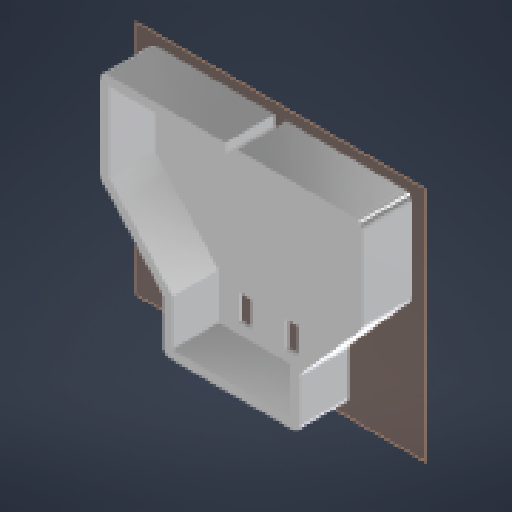
# Autodesk Inventor part: kracken Cover
Saved by Autodesk Inventor 2023 (Build 270158000, 158)
## iProperties
Created: 2024-02-18
Part Number: kracken Cover
Material: Aluminum 6061
Document SubType Name: Modeling
Designer: mavericks
Density: 2.7 g/cm^3
Appearance: Aluminum - Flat
Author: mavericks
Autodesk Inventor part; units mm, degrees
ref_plane "YZ Plane" through (0, 0, 0) normal (1, 0, 0) x (0, 1, 0)
ref_plane "XZ Plane" through (0, 0, 0) normal (0, 1, 0) x (-1, 0, 0)
ref_plane "Work Plane1" through (0, 0, -5.08) normal (0, 0, 1) x (1, 0, 0)
sketch "Sketch1" plane through (0, 0, -5.08) normal (0, 0, 1) x (1, 0, 0)
  line L0 (20.772, 33.401) -> (20.772, 19.8332)
  line L1 (20.772, 33.401) -> (1.011, 33.401)
  line L2 (1.011, 33.401) -> (1.011, 27.686)
  line L3 (1.011, 27.686) -> (-1.011, 27.686)
  line L4 (-1.011, 27.686) -> (-1.011, 33.401)
  line L5 (-1.011, 33.401) -> (-20.772, 33.401)
  line L6 (-20.772, 33.401) -> (-20.772, 19.8332)
  line L7 (-20.772, 19.8332) -> (-10.033, 7.78)
  line L8 (-10.033, 7.78) -> (-10.033, 0)
  line L9 (-10.033, 0) -> (10.033, 0)
  line L10 (10.033, 0) -> (10.033, 7.78)
  line L11 (10.033, 7.78) -> (20.772, 19.8332)
  line L12 (-22.3595, 34.9885) -> (-0.5765, 34.9885)
  line L13 (-0.5765, 34.9885) -> (22.3595, 34.9885)
  line L14 (22.3595, 34.9885) -> (22.3595, 19.2286)
  line L15 (22.3595, 19.2286) -> (11.6205, 7.1754)
  line L16 (11.6205, 7.1754) -> (11.6205, -1.5875)
  line L17 (11.6205, -1.5875) -> (-11.6205, -1.5875)
  line L18 (-11.6205, -1.5875) -> (-11.6205, 7.1754)
  line L19 (-11.6205, 7.1754) -> (-22.3595, 19.2286)
  line L20 (-22.3595, 19.2286) -> (-22.3595, 34.9885)
  point P0 (0, 0)
  point P1 (0, 0)
  point P2 (0, 27.686)
  point P3 (0, 0)
  dimension "d1" = 41.544
  dimension "d2" = 19.761
  dimension "d3" = 19.761
  dimension "d6" = 20.066
  dimension "d7" = 138.3
  dimension "d8" = 138.3
  dimension "d9" = 33.401
  dimension "d10" = 5.715
  dimension "d11" = 25.621
  dimension "d12" = 1.5875
  constraints: 42 end point, 9 perpendicular, 4 coincident, 2 midpoint, 2 point on line, 1 horizontal, 1 horizontal alignment, 1 vertical, 1 vertical alignment, 8 other
  measures "d1" distance between parallel lines of L0 L6
  measures "d2" distance of L4.end L5.end
  measures "d3" distance of L0.start L1.end
  measures "d6" distance of L8.end L9.end
  measures "d7" angle of L7 L6
  measures "d8" angle of L11 L0
  measures "d9" distance between parallel lines of L9 L5
  measures "d10" distance between parallel lines of L3 L5
  measures "d11" distance from line of L7.end L5
  measures "d12" distance between parallel lines of L5 L12
extrude "Extrusion1" add sketch "Sketch1" along normal blind 8.382
extrude "Extrusion2" add sketch "Sketch1" along normal blind 0.508 contours L0 L11 L10 L9 L8 L7 L6 L5 L4 L3 L2 L1
sketch "Sketch2" plane through (0, 0, 3.302) normal (0, 0, 1) x (1, 0, 0)
  line L0 (-22.3595, 34.9885) -> (22.3595, 34.9885) construction
  line L1 (-1.011, 27.686) -> (1.011, 27.686)
  line L2 (1.011, 27.686) -> (1.011, 34.9885)
  line L3 (1.011, 34.9885) -> (-1.011, 34.9885)
  line L4 (-1.011, 34.9885) -> (-1.011, 27.686)
  point P0 (0, 0)
  constraints: 8 end point, 2 parallel, 1 horizontal, 1 perpendicular, 1 point on line
extrude "Extrusion3" cut sketch "Sketch2" against normal through all
fillet "Fillet1" radius 1.27 8 edges at (-22.3595, 34.9885, -0.889) (-22.3595, 19.2286, -0.889) (-11.6205, 7.1754, -0.889) (-11.6205, -1.5875, -0.889) (11.6205, -1.5875, -0.889) (11.6205, 7.1754, -0.889) (22.3595, 19.2286, -0.889) (22.3595, 34.9885, -0.889)
sketch "Sketch4" plane through (0, 0, -5.08) normal (0, 0, -1) x (-1, 0, 0)
  circle A0 centre (-14.2442, 29.337) radius 1.8288 construction
  circle A1 centre (14.2546, 29.337) radius 1.8288 construction
  circle A2 centre (-14.2442, 29.337) radius 3.81
  circle A3 centre (14.2546, 29.337) radius 3.81
  line L0 (-1.8894, 5.6982) -> (-2.9308, 5.6982) construction
  line L1 (-2.9308, 2.3282) -> (-2.9308, 5.6982) construction
  line L2 (-2.9308, 2.3282) -> (-1.8894, 2.3282) construction
  line L3 (-1.8894, 5.6982) -> (-1.8894, 2.3282) construction
  line L4 (6.0354, 5.6982) -> (4.994, 5.6982) construction
  line L5 (4.994, 2.3282) -> (4.994, 5.6982) construction
  line L6 (4.994, 2.3282) -> (6.0354, 2.3282) construction
  line L7 (6.0354, 5.6982) -> (6.0354, 2.3282) construction
  line L8 (-1.3814, 1.8202) -> (-3.4388, 1.8202)
  line L9 (-3.4388, 1.8202) -> (-3.4388, 6.2062)
  line L10 (-3.4388, 6.2062) -> (-1.3814, 6.2062)
  line L11 (-1.3814, 6.2062) -> (-1.3814, 1.8202)
  line L12 (4.486, 6.2062) -> (6.5434, 6.2062)
  line L13 (6.5434, 6.2062) -> (6.5434, 1.8202)
  line L14 (6.5434, 1.8202) -> (4.486, 1.8202)
  line L15 (4.486, 1.8202) -> (4.486, 6.2062)
  point P0 (0, 0)
  dimension "d30" = 7.62
  dimension "d33" = 0.508
  dimension "d34" = 0.508
  constraints: 16 end point, 2 centre point, 2 coincident, 1 equal radius, 6 other
  measures "d30" diameter of A2
  measures "d33" distance between parallel lines of L3 L11
  measures "d34" distance between parallel lines of L5 L15
extrude "Extrusion4" cut sketch "Sketch4" against normal blind 25.4
equation "\"d3\" = d2"
equation "\"d8\" = d7"
body "Solid1"
